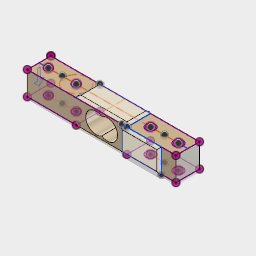
Load Cell 5kg YZC-133 v8 (Autodesk Fusion 360 design; units mm, degrees)
Autodesk Fusion 360 part; units mm, degrees
note: some values were not read from the file. Set by a fixed rule: which sketch regions a step uses.
sketch "Screw Holes" plane through (0, 0, 0) normal (0, 1, 0) x (1, 0, 0)
  line L0 (0, 0) -> (80, 0)
  line L1 (80, 0) -> (80, -12.7)
  line L2 (80, -12.7) -> (0, -12.7)
  line L3 (0, -12.7) -> (0, 0)
  line L4 (0, -6.35) -> (80, -6.35) construction
  circle A0 centre (5, -6.35) radius 2
  circle A1 centre (20, -6.35) radius 2
  circle A2 centre (60, -6.35) radius 2.5
  circle A3 centre (75, -6.35) radius 2.5
  line L5 (5, -6.35) -> (0, -6.35)
  line L6 (75, -6.35) -> (80, -6.35)
  line L7 (5, -6.35) -> (20, -6.35) construction
  line L8 (60, -6.35) -> (75, -6.35) construction
  point P0 (67.5, -6.35)
  point P1 (12.5, -6.35)
  dimension "d1" = 80
  dimension "d2" = 12.7
  dimension "d3" = 4
  dimension "d4" = 4
  dimension "d5" = 5
  dimension "d6" = 5
  dimension "d7" = 40
  dimension "d8" = 15
  dimension "d9" = 15
  measures "d1" distance of L0.start L0.end
  measures "d2" distance of L0.start L2.end
  measures "d3" diameter of A0
  measures "d4" diameter of A1
  measures "d5" diameter of A2
  measures "d6" diameter of A3
  measures "d7" distance of A1.centre A2.centre
  measures "d8" distance of A0.centre A1.centre
  measures "d9" distance of A2.centre A3.centre
extrude "Extrude1" add sketch "Screw Holes" against normal blind 12.7 contours L0 L1 L2 L3 | A0 | A1 | A2 | A3
extrude "Extrude2" cut sketch "Screw Holes" against normal through all contours A0 | A1 | A2 | A3
sketch "Loadcell Holes" plane through (0, 0, 12.7) normal (0, 0, 1) x (1, 0, 0)
  line L0 (80, 0) -> (0, 0)
  line L1 (0, 0) -> (0, -12.7)
  line L2 (0, -12.7) -> (80, -12.7)
  line L3 (80, -12.7) -> (80, 0)
  line L4 (40, -12.7) -> (40, 0) construction
  line L5 (0, -6.35) -> (80, -6.35) construction
  circle A0 centre (36.936, -6.35) radius 5.4886
  circle A1 centre (43.064, -6.35) radius 5.4886
  line L6 (36.936, -6.35) -> (43.064, -6.35)
extrude "Extrude3" cut sketch "Loadcell Holes" against normal blind 25 contours A0 A1 L6 | A0 A1 | A0 A1 L6 | A0 A1
sketch "Arrow" plane through (0, 0, 0) normal (-1, 0, 0) x (0, 0, 1)
  line L0 (12.7, 0) -> (0, 0)
  line L1 (0, 0) -> (0, -12.7)
  line L2 (0, -12.7) -> (12.7, -12.7)
  line L3 (12.7, -12.7) -> (12.7, 0)
  line L4 (5.511, -2.3504) -> (7.189, -2.3504)
  line L5 (7.189, -2.3504) -> (7.189, -8.0971)
  line L6 (7.189, -8.0971) -> (9.0409, -8.0971)
  line L7 (9.0409, -8.0971) -> (6.35, -10.7879)
  line L8 (6.35, -10.7879) -> (3.6591, -8.0971)
  line L9 (3.6591, -8.0971) -> (5.511, -8.0971)
  line L10 (5.511, -8.0971) -> (5.511, -2.3504)
  line L11 (6.35, -12.7) -> (6.35, 0) construction
  dimension "d20" = 45
  measures "d20" angle of L6 L7
extrude "Extrude4" cut sketch "Arrow" against normal blind 0.25 contours L4 L5 L6 L7 L8 L9 L10
sketch "Sketch5" plane through (0, 0, 0) normal (0, 1, 0) x (1, 0, 0)
  circle A0 centre (20, -6.35) radius 2
  circle A1 centre (60, -6.35) radius 2.5
  circle A2 centre (5, -6.35) radius 2
  circle A3 centre (75, -6.35) radius 2.5
  line L0 (80, -12.7) -> (80, 0)
  line L1 (80, 0) -> (0, 0)
  line L2 (0, 0) -> (0, -12.7)
  line L3 (0, -12.7) -> (80, -12.7)
  line L4 (40, 0) -> (40, -12.7) construction
  line L5 (26.35, 0) -> (53.65, 0)
  line L6 (53.65, 0) -> (53.65, -12.7)
  line L7 (53.65, -12.7) -> (26.35, -12.7)
  line L8 (26.35, -12.7) -> (26.35, 0)
  line L9 (26.35, -6.35) -> (40, -6.35) construction
  line L10 (40, -6.35) -> (53.65, -6.35) construction
  circle A4 centre (20, -6.35) radius 6.35 construction
extrude "Extrude6" add sketch "Sketch5" along normal blind 1.25 contours L1 L3 L5 L6 L7 L8
fillet "Fillet1" radius 1.25 4 edges at (26.35, 1.25, 6.35) (40, 1.25, 12.7) (53.65, 1.25, 6.35) (40, 1.25, 0)
sketch "Sketch6" plane through (0, -12.7, 0) normal (0, -1, 0) x (1, 0, 0)
  line L0 (80, 0) -> (80, 12.7)
  line L1 (80, 12.7) -> (0, 12.7)
  line L2 (0, 12.7) -> (0, 0)
  line L3 (0, 0) -> (80, 0)
  line L4 (26.35, 12.7) -> (26.35, 0)
  line L5 (26.35, 0) -> (0, 0)
  line L6 (0, 0) -> (0, 12.7)
  line L7 (0, 12.7) -> (26.35, 12.7)
  circle A0 centre (20, 6.35) radius 2
  circle A1 centre (5, 6.35) radius 2
  line L8 (53.65, 0) -> (53.65, 12.7)
  line L9 (53.65, 12.7) -> (80, 12.7)
  line L10 (80, 12.7) -> (80, 0)
  line L11 (80, 0) -> (53.65, 0)
  circle A2 centre (75, 6.35) radius 2.5
  circle A3 centre (60, 6.35) radius 2.5
  circle A4 centre (20, 6.35) radius 2
  circle A5 centre (60, 6.35) radius 2.5
  circle A6 centre (5, 6.35) radius 2
  circle A7 centre (75, 6.35) radius 2.5
  line L12 (5, 6.35) -> (20, 6.35) construction
  line L13 (60, 6.35) -> (75, 6.35) construction
  point P0 (67.5, 6.35)
  point P1 (12.5, 6.35)
extrude "Extrude7" add sketch "Sketch6" along normal blind 1.25 contours L1 L3 L4 L8
fillet "Fillet2" radius 1.25 4 edges at (26.35, -13.95, 6.35) (40, -13.95, 0) (53.65, -13.95, 6.35) (40, -13.95, 12.7)
sketch "Sketch7" plane through (0, 0, 12.7) normal (0, 0, 1) x (1, 0, 0)
  line L0 (26.35, -12.7) -> (53.65, -12.7)
  line L1 (53.65, -12.7) -> (80, -12.7)
  line L2 (80, -12.7) -> (80, 0)
  line L3 (80, 0) -> (53.65, 0)
  line L4 (53.65, 0) -> (26.35, 0)
  line L5 (26.35, 0) -> (0, 0)
  line L6 (0, 0) -> (0, -12.7)
  line L7 (0, -12.7) -> (26.35, -12.7)
  arc A0 (40, -1.7962) -> (40, -10.9038) centre (36.936, -6.35) ccw
  arc A1 (40, -10.9038) -> (40, -1.7962) centre (43.064, -6.35) ccw
  line L8 (51, 0) -> (72.1962, 0)
  line L9 (72.1962, 0) -> (72.1962, -12.7)
  line L10 (72.1962, -12.7) -> (51, -12.7)
  line L11 (51, -12.7) -> (51, 0)
extrude "Extrude8" add sketch "Sketch7" along normal blind 1.25 contours L0 L1 L3 L4 L8 L9 L10 L11
fillet "Fillet3" radius 1.25 4 edges at (51, -6.35, 13.95) (61.5981, 0, 13.95) (72.1962, -6.35, 13.95) (61.5981, -12.7, 13.95)
ref_plane "WorkPlane1" through (40, -6.975, 6.35) normal (0, 0, 1) x (-1, 0, 0)
ref_plane "WorkPlane2" through (65.5, -6.35, 6.975) normal (0, 1, 0) x (1, 0, 0)
ref_plane "WorkPlane3" through (40, -6.35, 6.35) normal (-1, 0, 0) x (0, 0, -1)
